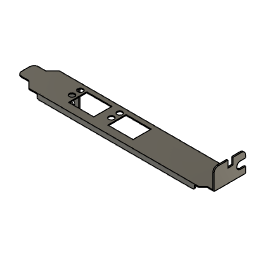
HPE P408i-p Fan Duct (Autodesk Fusion 360 archive; units mm, degrees)
design "X520-DA2 Full-Length Bracket"
Autodesk Fusion 360 part; units mm, degrees
sketch "Face" plane through (0, 0, 0) normal (0, 0, 1) x (1, 0, 0)
  line L0 (0, 0) -> (120.02, 0) construction
  line L1 (120.02, 0) -> (120.02, 21.59) construction
  line L2 (120.02, 21.59) -> (0, 21.59) construction
  line L3 (0, 21.59) -> (0, 6.655) construction
  line L4 (120.02, 2.54) -> (116.52, 2.54)
  line L5 (120.02, 21.59) -> (116.52, 21.59)
  line L6 (116.52, 2.54) -> (113.98, 0)
  line L7 (116.52, 2.54) -> (120.1121, 2.54) construction
  line L8 (116.52, 21.59) -> (113.35, 18.42)
  line L9 (116.52, 21.59) -> (120.02, 21.59) construction
  line L10 (113.35, 18.42) -> (11.1657, 18.42)
  line L11 (11.1657, 0) -> (7.0507, 4.115)
  line L12 (11.1657, 0) -> (18.2593, 0) construction
  line L13 (11.1657, 18.42) -> (7.0507, 14.305)
  line L14 (11.1657, 18.42) -> (18.3401, 18.42) construction
  line L15 (7.24, 21.59) -> (7.24, 0) construction
  line L16 (0, 9.21) -> (7.24, 9.21) construction
  line L17 (0, 9.21) -> (0, 14.305) construction
  line L18 (0, 9.21) -> (0, 4.115) construction
  line L19 (2.54, 14.305) -> (7.0507, 14.305)
  line L20 (2.54, 4.115) -> (7.0507, 4.115)
  line L21 (0, 9.21) -> (13.01, 9.21) construction
  line L22 (11.1657, 0) -> (113.98, 0)
  line L23 (120.02, 21.59) -> (120.02, 2.54)
  arc A0 (2.54, 14.305) -> (0, 11.765) centre (2.54, 11.765) ccw
  arc A1 (0, 6.655) -> (2.54, 4.115) centre (2.54, 6.655) ccw
  line L24 (0, 11.765) -> (0, 6.655)
  line L25 (0, 9.21) -> (30.5, 9.21) construction
  line L26 (0, 9.21) -> (54.3, 9.21) construction
  line L27 (30.5, 0) -> (30.5, 21.59) construction
  line L28 (45.75, 0) -> (45.75, 21.59) construction
  line L29 (54.3, 9.21) -> (69.55, 9.21) construction
  line L30 (27.75, 18.42) -> (27.75, 0) construction
  line L31 (27.75, 14.62) -> (30.5, 14.62) construction
  circle A2 centre (27.75, 14.62) radius 1.625
  line L32 (27.75, 9.57) -> (30.5, 9.57) construction
  circle A3 centre (27.75, 9.57) radius 1.625
  line L33 (69.55, 9.21) -> (69.55, 18.42) construction
  line L34 (30.5, 18.42) -> (69.55, 18.42) construction
  line L35 (69.55, 18.42) -> (69.55, 15.72) construction
  line L36 (69.55, 15.72) -> (30.5, 15.72) construction
  line L37 (30.5, 15.72) -> (30.5, 18.42) construction
  line L38 (30.5, 15.72) -> (45.75, 15.72)
  line L39 (45.75, 15.72) -> (45.75, 4.72)
  line L40 (45.75, 4.72) -> (30.5, 4.72)
  line L41 (30.5, 4.72) -> (30.5, 15.72)
  line L42 (69.55, 15.72) -> (54.3, 15.72)
  line L43 (54.3, 15.72) -> (54.3, 4.72)
  line L44 (54.3, 4.72) -> (69.55, 4.72)
  line L45 (69.55, 4.72) -> (69.55, 15.72)
  circle A4 centre (51.55, 14.62) radius 1.625
  circle A5 centre (51.55, 9.57) radius 1.625
  dimension "d1" = 120.02
  dimension "d2" = 21.59
  dimension "d3" = 19.05
  dimension "d4" = 3.5
  dimension "d6" = 135
  dimension "d7" = 135
  dimension "d8" = 18.42
  dimension "d9" = 135
  dimension "d10" = 135
  dimension "d13" = 9.21
  dimension "d14" = 5.095
  dimension "d15" = 5.095
  dimension "d16" = 10.19
  dimension "d17" = 13.01
  dimension "d35" = 2.54
  dimension "d36" = 2.54
  dimension "d37" = 30.5
  dimension "d38" = 54.3
  dimension "d39" = 15.25
  dimension "d42" = 15.25
  dimension "d45" = 2.75
  dimension "d46" = 3.8
  dimension "d47" = 3.25
  dimension "d48" = 8.85
  dimension "d49" = 3.25
  dimension "d51" = 2.7
  dimension "d52" = 11
  dimension "d53" = 11
  dimension "d54" = 3.25
  dimension "d55" = 3.25
  constraint horizontal L0
  constraint vertical L1
  constraint horizontal L2
  constraint vertical L3
  constraint coincident L0.start origin
  constraint horizontal L7
  constraint coincident L0 L6.end
  constraint coincident L0 L11.start
  constraint horizontal L9
  constraint horizontal L10
  constraint horizontal L12
  constraint horizontal L14
  constraint coincident L2 L15.start
  constraint perpendicular L0 L15
  constraint coincident L0 L15.end
  constraint coincident L3 L16.start
  constraint coincident L15 L16.end
  constraint perpendicular L15 L16
  constraint perpendicular L16 L17
  constraint perpendicular L16 L18
  constraint perpendicular L15 L19
  constraint perpendicular L15 L20
  constraint perpendicular L17 L21
  constraint parallel L4 L5
  constraint perpendicular L7 L23
  constraint coincident L17.end L19
  constraint tangent L19 A0
  constraint coincident L0.start L3
  constraint coincident L18.end L20
  constraint tangent L3 A1
  constraint tangent L20 A1
  constraint tangent A1 L24
  constraint perpendicular L17 L25
  constraint perpendicular L17 L26
  constraint perpendicular L10 L27
  constraint coincident L2 L27.end
  constraint coincident L25.end L27
  constraint coincident L0 L27.start
  constraint parallel L26 L29
  constraint coincident L10 L30.start
  constraint coincident L22 L30.end
  constraint perpendicular L22 L30
  constraint coincident L30 L31.start
  constraint coincident L27 L31.end
  constraint perpendicular L27 L31
  constraint coincident L31.start A2.centre
  constraint horizontal L32
  constraint coincident L30 L32.start
  constraint coincident L32.start A3.centre
  constraint coincident L10 L33.end
  constraint perpendicular L10 L33
  constraint horizontal L34
  constraint vertical L35
  constraint horizontal L36
  constraint vertical L37
  constraint coincident L27 L34.start
  constraint coincident L10 L34.start
  constraint horizontal L38
  constraint vertical L39
  constraint horizontal L40
  constraint vertical L41
  constraint horizontal L42
  constraint vertical L43
  constraint horizontal L44
  constraint vertical L45
  measures "d1" distance of L0.start L0.end
  measures "d2" distance of L0.start L2.end
  measures "d3" distance of L1.end L4.start
  measures "d4" distance of L4.start L4.end
  measures "d6" angle of L6 L7
  measures "d7" angle of L8 L9
  measures "d8" distance of L11.start L10.end
  measures "d9" angle of L11 L12
  measures "d10" angle of L13 L14
  measures "d13" distance of L10 L16
  measures "d14" distance of L16.start L17.end
  measures "d15" distance of L16.start L18.end
  measures "d16" distance of L19 L20
  measures "d17" distance of L16.start L21.end
  measures "d35" radius of A0
  measures "d36" radius of A1
  measures "d37" distance of L16.start L25.end
  measures "d38" distance of L16.start L26.end
  measures "d42" distance of L26.end L29.end
  measures "d45" distance of L27 L30
  measures "d46" distance of L10 L31
  measures "d47" diameter of A2
  measures "d48" distance of L10 L32
  measures "d49" diameter of A3
  measures "d51" distance of L34.start L36.end
  measures "d52" distance of L36.end L40.end
  measures "d53" distance of L35.end L44.end
  measures "d54" diameter of A4
  measures "d55" diameter of A5
ref_plane "WorkPlane1" through (120.02, 0, 0) normal (1, 0, 0) x (0, 1, 0)
sketch "Arm" plane through (120.02, 0, 0) normal (1, 0, 0) x (0, 1, 0)
  line L0 (0, 0) -> (21.59, 0) construction
  line L1 (21.59, 0) -> (21.59, 12.23) construction
  line L2 (19.05, 12.23) -> (5.08, 12.23) construction
  line L3 (0, 12.23) -> (0, 0) construction
  line L4 (0, 0) -> (2.54, 0) construction
  line L5 (2.54, 0) -> (2.54, 11.43) construction
  line L6 (2.54, 11.43) -> (0, 11.43) construction
  line L7 (0, 11.43) -> (0, 0) construction
  line L8 (21.59, 12.23) -> (18.41, 12.23) construction
  line L9 (18.41, 12.23) -> (18.41, 0) construction
  line L10 (18.41, 5.88) -> (21.59, 5.88) construction
  line L11 (21.59, 5.88) -> (21.59, 12.23) construction
  line L12 (2.54, 9.69) -> (2.54, 0)
  line L13 (2.54, 0) -> (21.59, 0)
  line L14 (18.41, 8.09) -> (21.5902, 8.09)
  line L15 (18.41, 3.67) -> (21.594, 3.67)
  arc A0 (18.41, 8.09) -> (18.41, 3.67) centre (18.41, 5.88) ccw
  line L16 (2.54, 12.23) -> (10.92, 12.23) construction
  line L17 (10.92, 12.23) -> (10.92, 0) construction
  line L18 (10.92, 0) -> (2.54, 0) construction
  line L19 (2.54, 0) -> (2.54, 12.23) construction
  line L20 (10.92, 12.23) -> (13.97, 12.23) construction
  line L21 (13.97, 12.23) -> (13.97, 0) construction
  line L22 (13.97, 0) -> (10.92, 0) construction
  line L23 (10.92, 0) -> (10.92, 12.23) construction
  line L24 (21.5902, 8.09) -> (2.54, 8.09) construction
  line L25 (10.92, 8.09) -> (13.97, 8.09)
  line L26 (13.97, 8.09) -> (13.97, 12.23)
  line L27 (21.59, 12.23) -> (13.97, 12.23)
  line L28 (10.92, 12.23) -> (2.54, 12.23)
  line L29 (13.97, 8.09) -> (16.3602, 12.23)
  line L30 (13.97, 8.09) -> (18.4336, 8.09) construction
  line L31 (10.92, 8.09) -> (8.5298, 12.23)
  line L32 (10.92, 8.09) -> (15.5777, 8.09) construction
  line L33 (21.59, 0) -> (21.59, 3.67)
  line L34 (21.59, 8.09) -> (21.59, 9.69)
  arc A1 (21.59, 9.69) -> (19.05, 12.23) centre (19.05, 9.69) ccw
  arc A2 (5.08, 12.23) -> (2.54, 9.69) centre (5.08, 9.69) ccw
  line L35 (0, 0) -> (2.54, 0)
  line L36 (2.54, 0) -> (2.54, 0.8)
  line L37 (2.54, 0.8) -> (0, 0.8)
  line L38 (0, 0.8) -> (0, 0)
  line L39 (10.92, 8.09) -> (10.92, 12.23)
  line L40 (2.54, 0.8) -> (21.59, 0.8016) construction
  dimension "d20" = 21.59
  dimension "d21" = 12.23
  dimension "d22" = 2.54
  dimension "d23" = 3.18
  dimension "d24" = 6.35
  dimension "d25" = 4.42
  dimension "d26" = 8.38
  dimension "d27" = 3.05
  dimension "d28" = 60
  dimension "d29" = 120
  dimension "d30" = 2.54
  dimension "d31" = 2.54
  dimension "d32" = 2.54
  dimension "d33" = 0.8
  dimension "d34" = 11.43
  constraint horizontal L0
  constraint vertical L1
  constraint horizontal L2
  constraint vertical L3
  constraint coincident L0.start L3.end
  constraint horizontal L4
  constraint vertical L5
  constraint horizontal L6
  constraint vertical L7
  constraint horizontal L8
  constraint vertical L9
  constraint horizontal L10
  constraint vertical L11
  constraint coincident L10.start A0.centre
  constraint horizontal L27
  constraint vertical L12
  constraint horizontal L13
  constraint vertical L33
  constraint coincident L10.start L9
  constraint coincident L0 L9.end
  constraint horizontal L14
  constraint coincident L9 L14.start
  constraint horizontal L15
  constraint coincident L9 L15.start
  constraint horizontal L16
  constraint vertical L17
  constraint horizontal L18
  constraint vertical L19
  constraint horizontal L20
  constraint vertical L21
  constraint horizontal L22
  constraint vertical L23
  constraint coincident L12 L24.end
  constraint perpendicular L12 L24
  constraint horizontal L25
  constraint vertical L26
  constraint coincident L24 L25.start
  constraint coincident L23 L25.start
  constraint collinear L27 L28
  constraint horizontal L30
  constraint coincident L2 L29.end
  constraint horizontal L32
  constraint coincident L14 L34.start
  constraint collinear L33 L34
  constraint coincident L15 L33.end
  constraint coincident L1.end L34
  constraint coincident L1.end L2
  constraint tangent L34 A1
  constraint tangent L2 A1
  constraint coincident L3.start L2
  constraint coincident L16.start L12
  constraint tangent L2 A2
  constraint tangent L12 A2
  constraint horizontal L35
  constraint vertical L36
  constraint horizontal L37
  constraint vertical L38
  constraint coincident L2 L31.end
  constraint coincident L1 L40.end
  measures "d20" distance of L0.start L0.end
  measures "d21" distance of L0.start L3.start
  measures "d22" distance of L0.start L4.end
  measures "d23" distance of L1.end L8.end
  measures "d24" distance of L1.end L10.end
  measures "d25" diameter of A0
  measures "d26" distance of L16.start L16.end
  measures "d27" distance of L16.end L20.end
  measures "d28" angle of L29 L30
  measures "d29" angle of L31 L32
  measures "d30" radius of A1
  measures "d31" radius of A2
  measures "d32" distance of L0.start L4.end
  measures "d33" distance of L0.start L37.end
  measures "d34" distance of L2 L37
ref_plane "WorkPlane2" through (0, 18.42, 0) normal (0, 1, 0) x (0, 0, 1)
sketch "Tabs" plane through (0, 18.42, 0) normal (0, 1, 0) x (1, 0, 0)
  line L0 (0, 0) -> (23.75, 0) construction
  line L1 (23.75, 0) -> (23.75, 13.05) construction
  line L2 (22.5, 14.3) -> (17.5, 14.3) construction
  line L3 (0, 14.3) -> (0, 0) construction
  line L4 (23.75, 0) -> (16.25, 0)
  line L5 (16.25, 0) -> (16.25, 13.05)
  line L6 (16.25, 14.3) -> (22.5, 14.3)
  line L7 (23.75, 13.05) -> (23.75, 0)
  line L8 (70.75, 0) -> (70.75, 13.05)
  line L9 (72, 14.3) -> (77, 14.3)
  line L10 (78.25, 13.05) -> (78.25, 0)
  line L11 (78.25, 0) -> (70.75, 0)
  line L12 (16.25, 11.325) -> (23.75, 11.325) construction
  line L13 (0, 0) -> (120.02, 0)
  circle A0 centre (20, 11.325) radius 1.325
  circle A1 centre (74.5, 11.325) radius 1.325
  arc A2 (17.5, 14.3) -> (16.25, 13.05) centre (17.5, 13.05) ccw
  arc A3 (72, 14.3) -> (70.75, 13.05) centre (72, 13.05) ccw
  arc A4 (78.25, 13.05) -> (77, 14.3) centre (77, 13.05) ccw
  arc A5 (23.75, 13.05) -> (22.5, 14.3) centre (22.5, 13.05) ccw
  line L14 (23.75, 13.05) -> (23.75, 14.3) construction
  line L15 (22.5, 14.3) -> (23.75, 14.3) construction
  dimension "d57" = 23.75
  dimension "d58" = 14.3
  dimension "d59" = 7.5
  dimension "d60" = 7.5
  dimension "d62" = 54.5
  dimension "d63" = 85.75
  dimension "d64" = 11.325
  dimension "d65" = 2.65
  dimension "d66" = 2.65
  dimension "d67" = 1.25
  dimension "d69" = 1.25
  dimension "d70" = 1.25
  dimension "d79" = 1.25
  constraint horizontal L0
  constraint vertical L1
  constraint horizontal L2
  constraint vertical L3
  constraint coincident L0.start L3.end
  constraint horizontal L4
  constraint vertical L5
  constraint horizontal L6
  constraint vertical L7
  constraint horizontal L11
  constraint vertical L8
  constraint horizontal L9
  constraint vertical L10
  constraint coincident L5 L12.start
  constraint coincident L7 L12.end
  constraint perpendicular L7 L12
  constraint midpoint L12 A0.centre
  constraint coincident L6.start L5
  constraint coincident L3.start L2
  constraint tangent L5 A2
  constraint tangent L2 A2
  constraint tangent L8 A3
  constraint tangent L9 A3
  constraint tangent L9 A4
  constraint tangent L10 A4
  constraint tangent L7 A5
  constraint tangent L6 A5
  constraint tangent A5 L14
  constraint parallel L1 L14
  constraint tangent A5 L15
  constraint perpendicular L14 L15
  measures "d57" distance of L0.start L0.end
  measures "d58" distance of L0.start L3.start
  measures "d59" distance of L0.end L4.end
  measures "d60" distance of L8.start L10.end
  measures "d62" distance of L7 L10
  measures "d64" distance of L12 L13
  measures "d65" diameter of A0
  measures "d66" diameter of A1
  measures "d67" radius of A2
  measures "d69" radius of A3
  measures "d70" radius of A4
  measures "d79" radius of A5
extrude "Extrude1" add sketch "Face" along normal blind 0.5
extrude "Extrude2" add sketch "Arm" along normal blind 0.8 contours L12 L13 L14 L15 A0 L25 L27 L28 L29 L31 L33 L34 A1 A2 L36 | L28 L31 L39 | L26 L27 L29
extrude "Extrude3" add sketch "Tabs" against normal blind 0.8 contours L8 L9 L10 L11 L13 A3 A4
extrude "Extrude4" add sketch "Tabs" against normal blind 0.8 contours L4 L5 L6 L7 L13 A2 A5
sketch "Sketch5" plane through (0, 0, 0) normal (0, 1, 0) x (1, 0, 0)
  line L0 (0, 0) -> (113.98, 0) construction
  line L1 (113.98, 0) -> (113.98, 2.54) construction
  line L2 (113.98, 2.54) -> (0, 2.54) construction
  line L3 (0, 2.54) -> (0, 0) construction
  line L4 (11.166, 0) -> (11.166, 2.54) construction
  line L5 (16.246, 0) -> (16.246, 2) construction
  line L6 (111.44, 0) -> (111.44, 1.54) construction
  line L7 (16.246, 0) -> (111.44, 0)
  line L8 (111.44, 0) -> (111.44, 2.54)
  line L9 (110.44, 2.54) -> (17.246, 2.54)
  line L10 (16.246, 1.54) -> (16.246, 0)
  arc A0 (17.246, 2.54) -> (16.246, 1.54) centre (17.246, 1.54) ccw
  arc A1 (111.44, 1.54) -> (110.44, 2.54) centre (110.44, 1.54) ccw
  dimension "d86" = 113.98
  dimension "d87" = 2.54
  dimension "d88" = 11.166
  dimension "d89" = 5.08
  dimension "d90" = 2.54
  dimension "d91" = 1
  dimension "d92" = 1
  constraint horizontal L0
  constraint vertical L1
  constraint horizontal L2
  constraint vertical L3
  constraint coincident L0.start L3.end
  constraint coincident L0 L4.start
  constraint coincident L2 L4.end
  constraint perpendicular L2 L4
  constraint coincident L0 L5.start
  constraint perpendicular L0 L5
  constraint coincident L0 L6.start
  constraint coincident L2 L8.end
  constraint perpendicular L2 L6
  constraint horizontal L7
  constraint vertical L8
  constraint horizontal L9
  constraint vertical L10
  constraint tangent L9 A0
  constraint tangent L10 A0
  constraint coincident L8.end L9
  constraint coincident L8.end L6
  constraint tangent L9 A1
  constraint tangent L6 A1
  measures "d86" distance of L0.start L0.end
  measures "d87" distance of L0.start L2.end
  measures "d88" distance of L3 L4
  measures "d89" distance of L4 L5
  measures "d90" distance of L1 L6
  measures "d91" radius of A0
  measures "d92" radius of A1
extrude "Extrude5" add sketch "Sketch5" along normal blind 0.8
